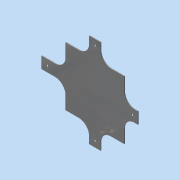
# Autodesk Inventor part: Bed Plate
Saved by Autodesk Inventor 2015 (Build 190159000, 159)
## iProperties
Created: 2016-06-24
Part Number: Bed Plate
Material: Generic
Document SubType Name: Modeling
Designer: Dustin
Density: 1 g/cm^3
Appearance: Default
Author: Dustin
Autodesk Inventor part; units mm, degrees
ref_plane "YZ Plane" through (0, 0, 0) normal (1, 0, 0) x (0, 1, 0)
sketch "Sketch1" plane through (0, 0, 0) normal (0, 0, 1) x (1, 0, 0)
  line L0 (0, 0) -> (300, 0)
  line L1 (300, 0) -> (300, 300)
  line L2 (300, 300) -> (0, 300)
  line L3 (0, 300) -> (0, 0)
  dimension "d0" = 300
  dimension "d1" = 300
  constraints: 8 end point, 2 parallel, 1 horizontal, 1 perpendicular
  measures "d0" distance of L2.end L0.start
  measures "d1" distance of L0.start L0.end
extrude "Extrusion1" add sketch "Sketch1" along normal blind 3.175
sketch "Sketch2" plane through (0, 0, 3.175) normal (0, 0, 1) x (1, 0, 0)
  line L0 (0, 300) -> (0, 0) projected
  line L1 (300, 300) -> (0, 300) projected
  line L2 (300, 0) -> (300, 300) projected
  line L3 (0, 0) -> (300, 0) projected
  point P0 (7, 293)
  point P1 (293, 293)
  point P2 (293, 7)
  point P3 (7, 7)
  dimension "d4" = 7
  dimension "d5" = 7
  dimension "d6" = 7
  dimension "d7" = 7
  dimension "d8" = 7
  dimension "d9" = 7
  dimension "d10" = 7
  dimension "d11" = 7
  measures "d4" distance from line of L0 point (7, 293)
  measures "d5" distance from line of L1 point (7, 293)
  measures "d6" distance from line of L2 point (293, 293)
  measures "d7" distance from line of L1 point (293, 293)
  measures "d8" distance from line of point (293, 7) L2
  measures "d9" distance from line of L3 point (293, 7)
  measures "d10" distance from line of L0 point (7, 7)
  measures "d11" distance from line of L3 point (7, 7)
hole "Hole1" at (7, 293, 3.175) at (293, 293, 3.175) at (293, 7, 3.175) at (7, 7, 3.175) direction (0, 0, -1) diameter 8 depth 25.4 tip angle 118
sketch "Sketch3" plane through (0, 0, 3.175) normal (0, 0, 1) x (1, 0, 0)
  line L0 (0, 300) -> (0, 0) projected
  line L1 (0, 0) -> (300, 0) projected
  line L2 (300, 0) -> (300, 300) projected
  point P0 (46, 254)
  point P1 (254, 254)
  point P2 (254, 46)
  point P3 (46, 46)
  dimension "d19" = 208
  dimension "d20" = 208
  dimension "d21" = 208
  dimension "d22" = 46
  dimension "d23" = 46
  dimension "d24" = 46
  dimension "d25" = 208
  dimension "d26" = 46
  measures "d19" distance of point (254, 254) point (46, 254)
  measures "d20" distance of point (46, 254) point (46, 46)
  measures "d21" distance of point (46, 46) point (254, 46)
  measures "d22" distance from line of L0 point (46, 46)
  measures "d23" distance from line of L1 point (46, 46)
  measures "d24" distance from line of L1 point (254, 46)
  measures "d25" distance of point (254, 46) point (254, 254)
  measures "d26" distance from line of L2 point (254, 254)
hole "Hole2" at (46, 254, 3.175) at (254, 254, 3.175) at (254, 46, 3.175) at (46, 46, 3.175) direction (0, 0, -1) diameter 3 depth 25.4 tip angle 118
sketch "Sketch4" plane through (0, 0, 3.175) normal (0, 0, 1) x (1, 0, 0)
  line L0 (0, 0) -> (300, 0) projected
  line L1 (0, 300) -> (0, 0) projected
  line L2 (300, 0) -> (300, 300) projected
  line L3 (300, 300) -> (0, 300) projected
  point P0 (293, 150)
  dimension "d38" = 7
  dimension "d41" = 150
  measures "d38" distance from line of L2 point (293, 150)
  measures "d41" distance from line of L0 point (293, 150)
hole "Hole3" at (293, 150, 3.175) direction (0, 0, -1) diameter 8 depth 25.4 tip angle 118
chamfer "Chamfer1" distance 75 angle 45 4 edges at (0, 0, 1.5875) (300, 0, 1.5875) (300, 300, 1.5875) (0, 300, 1.5875)
chamfer "Chamfer2" distance 53 angle 45 8 edges at (75, 0, 1.5875) (0, 75, 1.5875) (225, 0, 1.5875) (300, 75, 1.5875) (300, 225, 1.5875) (225, 300, 1.5875) (75, 300, 1.5875) (0, 225, 1.5875)
sketch "Sketch5" plane through (0, 0, 3.175) normal (0, 0, 1) x (1, 0, 0)
  circle A0 centre (293, 150) radius 4 projected
  circle A1 centre (254, 46) radius 1.5 projected
  circle A2 centre (46, 254) radius 1.5 projected
  circle A3 centre (254, 254) radius 1.5 projected
  circle A4 centre (46, 46) radius 1.5 projected
  line L0 (0, 172) -> (37.4767, 262.4767) projected
  line L1 (0, 172) -> (0, 128) projected
  line L2 (37.4767, 37.5233) -> (0, 128) projected
  line L3 (37.5233, 37.4767) -> (37.4767, 37.5233) projected
  line L4 (128, 0) -> (37.5233, 37.4767) projected
  line L5 (128, 0) -> (172, 0) projected
  line L6 (262.4767, 37.4767) -> (172, 0) projected
  line L7 (262.5233, 37.5233) -> (262.4767, 37.4767) projected
  line L8 (300, 128) -> (262.5233, 37.5233) projected
  line L9 (300, 128) -> (300, 172) projected
  line L10 (262.5233, 262.4767) -> (300, 172) projected
  line L11 (262.4767, 262.5233) -> (262.5233, 262.4767) projected
  line L12 (172, 300) -> (262.4767, 262.5233) projected
  line L13 (172, 300) -> (128, 300) projected
  line L14 (37.5233, 262.5233) -> (128, 300) projected
  line L15 (37.4767, 262.4767) -> (37.5233, 262.5233) projected
  line L16 (37.5233, 37.4767) -> (87.5233, 37.4767)
  arc A5 (128, 0) -> (87.5233, 37.4767) centre (87.5233, -3.1201) ccw
  line L17 (150, 0) -> (150, 20.8138)
  line L18 (262.4767, 37.4767) -> (212.4767, 37.4767)
  arc A6 (212.4767, 37.4767) -> (172, 0) centre (212.4767, -3.1201) ccw
  line L19 (262.5233, 37.5233) -> (262.5233, 87.5233)
  arc A7 (300, 128) -> (262.5233, 87.5233) centre (303.1201, 87.5233) ccw
  line L20 (262.5233, 262.4767) -> (262.5233, 212.4767)
  arc A8 (262.5233, 212.4767) -> (300, 172) centre (303.1201, 212.4767) ccw
  line L21 (262.4767, 262.5233) -> (212.4767, 262.5233)
  arc A9 (172, 300) -> (212.4767, 262.5233) centre (212.4767, 303.1201) ccw
  line L22 (37.5233, 262.5233) -> (87.5233, 262.5233)
  arc A10 (87.5233, 262.5233) -> (128, 300) centre (87.5233, 303.1201) ccw
  line L23 (37.4767, 262.4767) -> (37.4767, 212.4767)
  arc A11 (0, 172) -> (37.4767, 212.4767) centre (-3.1201, 212.4767) ccw
  line L24 (37.4767, 37.5233) -> (37.4767, 87.5233)
  arc A12 (37.4767, 87.5233) -> (0, 128) centre (-3.1201, 87.5233) ccw
  point P0 (0, 0)
  point P1 (150, 150)
  dimension "d56" = 50
  dimension "d57" = 150
  dimension "d58" = 150
  dimension "d61" = 360
  constraints: 18 end point, 16 point on circle, 8 centre point, 2 symmetric about line, 1 horizontal, 1 midpoint, 1 tangent, 1 vertical, 50 other
  measures "d56" distance of L3.start L16.end
  measures "d57" distance from line of L13 point (150, 150)
  measures "d58" distance from line of L1 point (150, 150)
extrude "Extrusion2" add sketch "Sketch5" along normal blind 25.4 contours L16 A5 L4 | A6 L18 L6
ref_plane "Work Plane1" through (37.4767, 37.5233, 28.575) normal (0, 0, 1) x (1, 0, 0)
sketch "Sketch6" plane through (37.4767, 37.5233, 28.575) normal (0, 0, 1) x (1, 0, 0)
  line L0 (-37.4767, 90.4767) -> (0, 0)
  line L1 (0, 0) -> (0, 50)
  arc A0 (0, 50) -> (-37.4767, 90.4767) centre (-40.5967, 50) ccw
  line L2 (0, 224.9533) -> (-37.4767, 134.4767)
  arc A1 (-37.4767, 134.4767) -> (0, 174.9533) centre (-40.5967, 174.9533) ccw
  line L3 (0, 174.9533) -> (0, 224.9533)
  line L4 (90.5233, 262.4767) -> (0.0467, 225)
  line L5 (0.0467, 225) -> (50.0467, 225)
  arc A2 (50.0467, 225) -> (90.5233, 262.4767) centre (50.0467, 265.5967) ccw
  line L6 (225, 225) -> (134.5233, 262.4767)
  line L7 (262.5233, 134.4767) -> (225.0467, 224.9533)
  line L8 (262.5233, 134.4767) -> (225.0467, 224.9533)
  line L9 (225.0467, 224.9533) -> (225.0467, 174.9533)
  arc A3 (225.0467, 174.9533) -> (262.5233, 134.4767) centre (265.6434, 174.9533) ccw
  line L10 (225.0467, 0) -> (262.5233, 90.4767)
  arc A4 (262.5233, 90.4767) -> (225.0467, 50) centre (265.6434, 50) ccw
  line L11 (225.0467, 50) -> (225.0467, 0)
  line L12 (134.5233, -37.5233) -> (225, -0.0467)
  line L13 (225, -0.0467) -> (175, -0.0467)
  arc A5 (175, -0.0467) -> (134.5233, -37.5233) centre (175, -40.6434) ccw
  line L14 (0.0467, -0.0467) -> (90.5233, -37.5233)
  arc A6 (90.5233, -37.5233) -> (50.0467, -0.0467) centre (50.0467, -40.6434) ccw
  line L15 (50.0467, -0.0467) -> (0.0467, -0.0467)
  point P0 (-37.4767, -37.5233)
extrude "Extrusion3" cut sketch "Sketch6" against normal through all
ref_plane "Work Plane2" through (212.4767, 262.5233, 28.575) normal (0, 0, 1) x (1, 0, 0)
sketch "Sketch7" plane through (212.4767, 262.5233, 28.575) normal (0, 0, 1) x (1, 0, 0)
  line L0 (50, 0) -> (-40.4767, 37.4767) projected
  arc A0 (-40.4767, 37.4767) -> (0, 0) centre (0, 40.5967) ccw projected
  line L1 (0, 0) -> (50, 0) projected
  point P0 (-212.4767, -262.5233)
extrude "Extrusion4" cut sketch "Sketch7" against normal through all
sketch "Sketch8" plane through (0, 128, 0) normal (-1, 0, 0) x (0, 0, 1)
  line L0 (0, 44) -> (3.175, 44) projected
  line L1 (0, 44) -> (0, 0) projected
  line L2 (3.175, 0) -> (0, 0) projected
  line L3 (3.175, 44) -> (3.175, 0) projected
  point P0 (0, -128)
extrude "Extrusion5" add sketch "Sketch8" along normal blind 40
sketch "Sketch9" plane through (0, 0, 3.175) normal (0, 0, 1) x (1, 0, 0)
  line L0 (0, 128) -> (-40, 128) projected
  line L1 (-40, 128) -> (-40, 172) projected
  point P0 (0, 0)
  point P1 (-33, 150)
  dimension "d81" = 22
  dimension "d82" = 7
  measures "d81" distance from line of L0 point (-33, 150)
  measures "d82" distance from line of L1 point (-33, 150)
hole "Hole5" at (-33, 150, 3.175) direction (0, 0, -1) diameter 8 depth 25.4 tip angle 118
sketch "Sketch10" plane through (128, 0, 0) normal (0, -1, 0) x (1, 0, 0)
  line L0 (44, 3.175) -> (44, 0) projected
  line L1 (0, 3.175) -> (44, 3.175) projected
  line L2 (0, 0) -> (0, 3.175) projected
  line L3 (0, 0) -> (44, 0) projected
  point P0 (-128, 0)
extrude "Extrusion6" add sketch "Sketch10" along normal blind 15
sketch "Sketch11" plane through (0, 0, 3.175) normal (0, 0, 1) x (1, 0, 0)
  line L0 (172, -15) -> (128, -15) projected
  point P0 (0, 0)
  point P1 (150, -8)
  dimension "d92" = 7
  dimension "d93" = 22
  measures "d92" distance from line of L0 point (150, -8)
  measures "d93" horizontal distance of L0.end point (150, -8)
hole "Hole6" at (150, -8, 3.175) direction (0, 0, -1) diameter 8 depth 25.4 tip angle 118
sketch "Sketch12" plane through (128, 300, 3.175) normal (0, 1, 0) x (1, 0, 0)
  line L0 (0, 0) -> (0, 3.175) projected
  line L1 (44, 0) -> (0, 0) projected
  line L2 (44, 3.175) -> (44, 0) projected
  line L3 (44, 3.175) -> (0, 3.175) projected
  point P0 (-128, 3.175)
extrude "Extrusion7" add sketch "Sketch12" along normal blind 15
sketch "Sketch13" plane through (0, 0, 3.175) normal (0, 0, 1) x (1, 0, 0)
  line L0 (172, 300) -> (172, 315) projected
  point P0 (0, 0)
  point P1 (150, 308)
  dimension "d103" = 22
  dimension "d104" = 7
  measures "d103" distance from line of L0 point (150, 308)
  measures "d104" vertical distance of L0.end point (150, 308)
hole "Hole7" at (150, 308, 3.175) direction (0, 0, -1) diameter 8 depth 25.4 tip angle 118
sketch "Sketch14" plane through (128, 315, 3.175) normal (0, 1, 0) x (1, 0, 0)
  line L0 (0, 3.175) -> (0, 0) projected
  line L1 (0, 0) -> (44, 0) projected
  line L2 (44, 0) -> (44, 3.175) projected
  line L3 (44, 3.175) -> (0, 3.175) projected
  point P0 (-128, 3.175)
extrude "Extrusion8" add sketch "Sketch14" along normal blind 15
sketch "Sketch15" plane through (300, 128, 0) normal (1, 0, 0) x (0, 0, -1)
  line L0 (-3.175, 44) -> (0, 44) projected
  line L1 (-3.175, 0) -> (-3.175, 44) projected
  line L2 (0, 0) -> (-3.175, 0) projected
  line L3 (0, 0) -> (0, 44) projected
  point P0 (0, -128)
extrude "Extrusion9" add sketch "Sketch15" along normal blind 15
sketch "Sketch16" plane through (128, -15, 0) normal (0, -1, 0) x (1, 0, 0)
  line L0 (44, 0) -> (44, 3.175) projected
  line L1 (44, 3.175) -> (0, 3.175) projected
  line L2 (0, 3.175) -> (0, 0) projected
  line L3 (0, 0) -> (44, 0) projected
  point P0 (-128, 0)
extrude "Extrusion10" add sketch "Sketch16" along normal blind 15
sketch "Sketch17" plane through (-40, 128, 0) normal (-1, 0, 0) x (0, 0, 1)
  line L0 (3.175, 44) -> (0, 44) projected
  line L1 (0, 44) -> (0, 0) projected
  line L2 (0, 0) -> (3.175, 0) projected
  line L3 (3.175, 0) -> (3.175, 44) projected
  point P0 (0, -128)
extrude "Extrusion11" add sketch "Sketch17" along normal blind 15
sketch "Sketch18" plane through (0, 0, 3.175) normal (0, 0, 1) x (1, 0, 0)
  circle A0 centre (-33, 150) radius 4 projected
  line L0 (0, 172) -> (-55, 172) projected
  point P0 (0, 0)
  point P1 (-41, 150)
  dimension "d120" = 8
  dimension "d121" = 22
  measures "d120" distance of A0.centre point (-41, 150)
  measures "d121" distance from line of L0 point (-41, 150)
hole "Hole8" at (-41, 150, 3.175) direction (0, 0, -1) diameter 3 depth 8 tip angle 118
pattern_circular "Circular Pattern2" count 4 over 360 about axis through (-33, 150, -9.525) along (0, 0, 1) of "Hole8"
sketch "Sketch19" plane through (0, 0, 3.175) normal (0, 0, 1) x (1, 0, 0)
  circle A0 centre (150, -8) radius 4 projected
  line L0 (128, 0) -> (128, -30) projected
  point P0 (0, 0)
  point P1 (150, -16)
  dimension "d132" = 8
  dimension "d133" = 22
  measures "d132" distance of A0.centre point (150, -16)
  measures "d133" distance from line of L0 point (150, -16)
hole "Hole9" at (150, -16, 3.175) direction (0, 0, -1) diameter 3 depth 8 tip angle 118
pattern_circular "Circular Pattern3" count 4 over 360 about axis through (150, -8, -9.525) along (0, 0, 1) of "Hole9"
sketch "Sketch20" plane through (0, 0, 3.175) normal (0, 0, 1) x (1, 0, 0)
  circle A0 centre (293, 150) radius 4 projected
  line L0 (300, 128) -> (315, 128) projected
  point P0 (0, 0)
  point P1 (301, 150)
  dimension "d144" = 8
  dimension "d145" = 22
  measures "d144" distance of A0.centre point (301, 150)
  measures "d145" distance from line of L0 point (301, 150)
hole "Hole10" at (301, 150, 3.175) direction (0, 0, -1) diameter 3 depth 8 tip angle 118
pattern_circular "Circular Pattern4" count 4 over 360 about axis through (293, 150, -9.525) along (0, 0, 1) of "Hole10"
sketch "Sketch21" plane through (0, 0, 3.175) normal (0, 0, 1) x (1, 0, 0)
  circle A0 centre (150, 308) radius 4 projected
  point P0 (0, 0)
  point P1 (150.192, 316)
  dimension "d156" = 8
  measures "d156" vertical distance of A0.centre point (150.192, 316)
hole "Hole11" at (150.192, 316, 3.175) direction (0, 0, -1) diameter 3 depth 8 tip angle 118
pattern_circular "Circular Pattern5" count 4 over 360 about axis through (150, 308, -9.525) along (0, 0, 1) of "Hole11"
body "Solid1"
